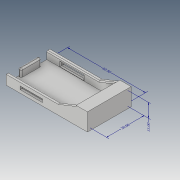
# Autodesk Inventor part: parte1
Saved by Autodesk Inventor 2019 (Build 230136000, 136)
## iProperties
Created: 2020-09-17
Part Number: parte1
Material: Generic
Document SubType Name: Modeling
Designer: giacomo
Density: 1 g/cm^3
Appearance: Default
Author: giacomo
Autodesk Inventor part; units mm, degrees
ref_plane "YZ Plane" through (0, 0, 0) normal (1, 0, 0) x (0, 1, 0)
ref_plane "XZ Plane" through (0, 0, 0) normal (0, 1, 0) x (-1, 0, 0)
ref_plane "XY Plane" through (0, 0, 0) normal (0, 0, 1) x (1, 0, 0)
sketch "Sketch1" plane through (0, 0, 0) normal (0, 1, 0) x (-1, 0, 0)
  line L0 (26.4044, 9.2294) -> (-30.5956, 9.2294) construction
  line L1 (-30.5956, 9.2294) -> (-30.5956, -17.7706) construction
  line L2 (-30.5956, -17.7706) -> (26.4044, -17.7706) construction
  line L3 (26.4044, -17.7706) -> (26.4044, 9.2294) construction
  point P0 (0, 0)
  dimension "d0" = 57
  dimension "d1" = 27
  constraints: 8 end point, 2 parallel, 1 horizontal, 1 perpendicular
  measures "d0" distance of L1.end L2.end
  measures "d1" distance of L0.end L1.end
sketch "Sketch2" plane through (0, 0, 0) normal (0, 1, 0) x (-1, 0, 0)
  line L0 (26.4044, -17.7706) -> (26.4044, 9.2294) construction
  line L1 (-30.5956, -17.7706) -> (26.4044, -17.7706) construction
  line L2 (-30.5956, 9.2294) -> (-30.5956, -17.7706) construction
  line L3 (26.4044, 9.2294) -> (-30.5956, 9.2294) construction
  line L4 (30.4044, 13.2294) -> (30.4044, -21.7706)
  line L5 (30.4044, -21.7706) -> (-34.5956, -21.7706)
  line L6 (-34.5956, -21.7706) -> (-34.5956, 13.2294)
  line L7 (-34.5956, 13.2294) -> (30.4044, 13.2294)
  point P0 (0, 0)
  dimension "d2" = 4
  constraints: 8 end point, 3 other
  measures "d2" distance between parallel lines of L0 L4
extrude "Extrusion1" add sketch "Sketch2" against normal blind 1.5
sketch "Sketch3" plane through (0, 0, 0) normal (0, 1, 0) x (1, 0, 0)
  line L0 (-30.4044, -13.2294) -> (-30.4044, 21.7706) projected
  line L1 (34.5956, -13.2294) -> (-30.4044, -13.2294) projected
  line L2 (34.5956, 21.7706) -> (34.5956, -13.2294) projected
  line L3 (-30.4044, 21.7706) -> (34.5956, 21.7706) projected
  line L4 (-27.9044, 12.2706) -> (-27.9044, -3.7294)
  line L5 (-26.4044, -10.7294) -> (32.0956, -10.7294)
  line L6 (32.0956, -10.7294) -> (32.0956, 19.2706)
  line L7 (32.0956, 19.2706) -> (-28.4044, 19.2706)
  line L8 (-26.4044, -10.7294) -> (-30.4044, -10.7294)
  line L9 (-28.4044, 19.2706) -> (-30.4044, 19.2706)
  line L10 (-30.4044, -13.2294) -> (-30.4044, 21.7706) projected
  line L11 (-27.9044, -3.7294) -> (-30.4044, -3.7294)
  line L12 (-27.9044, 12.2706) -> (-30.4044, 12.2706)
  point P0 (0, 0)
  dimension "d5" = 2.5
  dimension "d6" = 7
  dimension "d7" = 7
  dimension "d35" = 2.5
  constraints: 16 end point, 4 point on line, 3 perpendicular, 1 parallel, 2 other
  measures "d5" distance between parallel lines of L0 L4
  measures "d6" distance between parallel lines of L8 L11
  measures "d7" distance between parallel lines of L12 L9
  measures "d35" distance between parallel lines of L5 L1
extrude "Extrusion2" add sketch "Sketch3" along normal blind 6 contours L0 L8 L5 L6 L7 L9 L3 L2 L1 | L0 L12 L4 L11
sketch "Sketch4" plane through (-30.4044, -1.5, 13.2294) normal (0, 0, 1) x (1, 0, 0)
  line L0 (0, 7.5) -> (65, 7.5) projected
  line L1 (65, 7.5) -> (65, 12.5)
  line L2 (65, 12.5) -> (65, 14)
  line L3 (65, 14) -> (58, 14)
  line L4 (58, 14) -> (41.6092, 7.5)
  line L5 (41.6092, 7.5) -> (65, 7.5)
  line L6 (0, 7.5) -> (62.5, 7.5) projected
  point P0 (30.4044, 1.5)
  point P1 (49.8046, 7.5)
  point P2 (58, 7.5)
  dimension "d10" = 5
  dimension "d11" = 1.5
  dimension "d12" = 7
  constraints: 10 end point, 4 point on line, 1 collinear, 1 perpendicular, 1 vertical
  measures "d10" distance of L0.end L1.end
  measures "d11" distance of L1.end L2.end
  measures "d12" distance of L2.end L3.end
extrude "Extrusion3" add sketch "Sketch4" against normal up to surface (2.5 mm away)
extrude "Extrusion4" add sketch "Sketch4" against normal up to surface (2.5 mm away) from surface at -32.5
sketch "Sketch5" plane through (34.5956, -1.5, 13.2294) normal (1, 0, 0) x (0, 0, -1)
  line L0 (0, 14) -> (2.5, 14) projected
  line L1 (2.5, 7.5) -> (32.5, 7.5) projected
  line L2 (2.5, 14) -> (32.5, 14)
  line L3 (32.5, 14) -> (32.5, 7.5)
  line L4 (32.5, 7.5) -> (2.5, 7.5)
  line L5 (2.5, 7.5) -> (2.5, 14)
  point P0 (13.2294, 1.5)
  constraints: 8 end point, 2 parallel, 1 horizontal, 1 perpendicular
extrude "Extrusion5" add sketch "Sketch5" against normal up to surface (2.5 mm away)
sketch "Sketch6" plane through (27.5956, 12.5, 13.2294) normal (0, 1, 0) x (1, 0, 0)
  line L0 (7, 35) -> (0, 35) projected
  line L1 (0, 0) -> (-16.3908, 0) projected
  line L2 (7, 35) -> (-2, 35)
  line L3 (-2, 35) -> (-2, 0)
  line L4 (-2, 0) -> (7, 0)
  line L5 (7, 0) -> (7, 35)
  point P0 (-27.5956, 13.2294)
  point P1 (4.5, 32.5)
  dimension "d21" = 9
  constraints: 8 end point, 2 parallel, 1 horizontal, 1 perpendicular, 1 point on line
  measures "d21" distance of L4.end L3.end
extrude "Extrusion6" add sketch "Sketch6" against normal blind 1.5
sketch "Sketch7" plane through (-30.4044, -1.5, 13.2294) normal (0, 0, 1) x (1, 0, 0)
  line L0 (11.1606, 5) -> (29.1606, 5)
  line L1 (29.1606, 5) -> (29.1606, 2.5)
  line L2 (29.1606, 2.5) -> (11.1606, 2.5)
  line L3 (11.1606, 2.5) -> (11.1606, 5)
  line L4 (65, 0) -> (0, 0) projected
  point P0 (30.4044, 1.5)
  dimension "d22" = 18
  dimension "d23" = 2.5
  dimension "d36" = 2.5
  constraints: 8 end point, 2 parallel, 1 horizontal, 1 perpendicular
  measures "d22" distance of L0.start L0.end
  measures "d23" distance of L0.end L1.end
  measures "d36" distance between parallel lines of L4 L2
extrude "Extrusion7" cut sketch "Sketch7" against normal through all
fillet "Fillet1" radius 1 8 edges at (-27.9044, 3, 3.7294) (-27.9044, 6, -4.2706) (-27.9044, 3, -12.2706) (-30.4044, 6, -4.2706) (-29.1544, 6, 3.7294) (-30.4044, 3, -12.2706) (-29.1544, 6, -12.2706) (-30.4044, 3, 3.7294)
fillet "Fillet2" radius 0.8 13 edges at (18.4002, 8.8534, 10.7294) (-9.5998, 6, 10.7294) (-9.5998, 6, -19.2706) (18.4002, 8.8534, -19.2706) (25.5956, 11, -4.2706) (-10.2438, 3.5, -19.2706) (-10.2438, 1, -19.2706) (-10.2438, 3.5, 10.7294) (-10.2438, 1, 10.7294) (-19.2438, 2.25, 10.7294) (-1.2438, 2.25, 10.7294) (-1.2438, 2.25, -19.2706) (-19.2438, 2.25, -19.2706)
body "Solid1"
